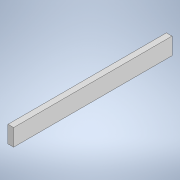
# Autodesk Inventor part: body_1
Saved by Autodesk Inventor 2021 (Build 250183000, 183)
## iProperties
Created: 2021-02-20
Part Number: body_1
Material: Generic
Document SubType Name: Modeling
Designer: bagal
Density: 1 g/cm^3
Appearance: Default
Author: bagal
Autodesk Inventor part; units mm, degrees
ref_plane "YZ Plane" through (0, 0, 0) normal (1, 0, 0) x (0, 1, 0)
ref_plane "XZ Plane" through (0, 0, 0) normal (0, 1, 0) x (-1, 0, 0)
ref_plane "XY Plane" through (0, 0, 0) normal (0, 0, 1) x (1, 0, 0)
sketch "Sketch1" plane through (0, 0, 0) normal (1, 0, 0) x (0, 1, 0)
  line L0 (5.1481, 16.1163) -> (5.1481, -161.6837)
  line L1 (5.1481, -161.6837) -> (-13.9019, -161.6837)
  line L2 (-13.9019, -161.6837) -> (-13.9019, 16.1163)
  line L3 (-13.9019, 16.1163) -> (5.1481, 16.1163)
  point P0 (0, 0)
  dimension "d0" = 177.8
  dimension "d1" = 19.05
  dimension "d2" = 177.8
  constraints: 8 end point, 1 horizontal, 1 perpendicular, 1 vertical
  measures "d0" distance of L0.start L0.end
  measures "d1" distance of L0.end L1.end
  measures "d2" distance of L1.end L2.end
extrude "Extrusion1" add sketch "Sketch1" along normal blind 6.35
body "Solid1"
